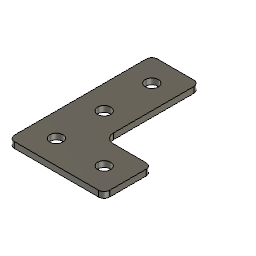
1-008 L Bracket Flat Plate SHORT v4 (Autodesk Fusion 360 design; units mm, degrees)
Autodesk Fusion 360 part; units mm, degrees
sketch "Sketch1" plane through (0, 0, 0) normal (0, 0, 1) x (1, 0, 0)
  line L0 (0, 0) -> (50.8, 0)
  line L1 (50.8, 0) -> (50.8, 25.4)
  line L2 (50.8, 25.4) -> (25.4, 25.4)
  line L3 (25.4, 25.4) -> (25.4, 76.2)
  line L4 (25.4, 76.2) -> (0, 76.2)
  line L5 (0, 76.2) -> (0, 0)
  line L6 (0, 0) -> (25.4, 25.4) construction
  circle A0 centre (12.7, 12.7) radius 3.429
  circle A1 centre (38.1, 12.7) radius 3.429
  circle A2 centre (12.7, 38.1) radius 3.429
  circle A3 centre (12.7, 63.5) radius 3.429
  dimension "d1" = 25.4
  dimension "d2" = 25.4
  dimension "d3" = 50.8
  dimension "d4" = 76.2
  dimension "d5" = 6.858
  dimension "d6" = 25.4
  dimension "d7" = 25.4
  dimension "d8" = 25.4
  dimension "d9" = 12.7
  constraint coincident L0.start L5.end
  constraint horizontal L0
  constraint perpendicular L0 L1
  constraint perpendicular L1 L2
  constraint perpendicular L2 L3
  constraint perpendicular L3 L4
  constraint perpendicular L0 L5
  constraint midpoint L6 A0.centre
  constraint vertical A2.centre A3.centre
  constraint vertical A0.centre A2.centre
  constraint horizontal A0.centre A1.centre
  constraint equal A0 A1
  constraint equal A0 A2
  constraint equal A2 A3
  measures "d1" distance of L0.end L1.end
  measures "d2" distance of L3.end L4.end
  measures "d3" distance of L1 L5
  measures "d4" distance of L0 L4
  measures "d5" diameter of A1
  measures "d6" distance of A0.centre A1.centre
  measures "d7" distance of A0.centre A2.centre
  measures "d8" distance of A2.centre A3.centre
  measures "d9" distance of L4 A3.centre
extrude "Extrude1" add sketch "Sketch1" along normal blind 3.175
fillet "Fillet1" radius 3 5 edges at (0, 0, 1.5875) (50.8, 0, 1.5875) (50.8, 25.4, 1.5875) (0, 76.2, 1.5875) (25.4, 76.2, 1.5875)
fillet "Fillet1" radius 5 1 edges at (25.4, 25.4, 1.5875)
sketch "DXF" plane through (0, 0, 3.175) normal (0, 0, 1) x (-1, 0, 0)
  arc A0 (-25.4, -73.2) -> (-22.4, -76.2) centre (-22.4, -73.2) ccw
  line L0 (-22.4, -76.2) -> (-3, -76.2)
  arc A1 (-3, -76.2) -> (0, -73.2) centre (-3, -73.2) ccw
  line L1 (0, -73.2) -> (0, -3)
  arc A2 (0, -3) -> (-3, 0) centre (-3, -3) ccw
  line L2 (-3, 0) -> (-47.8, 0)
  arc A3 (-47.8, 0) -> (-50.8, -3) centre (-47.8, -3) ccw
  line L3 (-50.8, -3) -> (-50.8, -22.4)
  arc A4 (-50.8, -22.4) -> (-47.8, -25.4) centre (-47.8, -22.4) ccw
  line L4 (-47.8, -25.4) -> (-30.4, -25.4)
  arc A5 (-25.4, -30.4) -> (-30.4, -25.4) centre (-30.4, -30.4) ccw
  line L5 (-25.4, -30.4) -> (-25.4, -73.2)
  circle A6 centre (-12.7, -63.5) radius 3.429
  circle A7 centre (-12.7, -12.7) radius 3.429
  circle A8 centre (-12.7, -38.1) radius 3.429
  circle A9 centre (-38.1, -12.7) radius 3.429
equation "d10 = ( 1 / 8 ) * 1 in"
